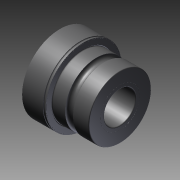
# Autodesk Inventor part: NKXZ12
Saved by Autodesk Inventor 2011 SP1 (Build 150282100, 282)
## iProperties
Created: 2016-11-09
Part Number: NKXZ12
Catalog Web Link: www.cadenas.de
Description: NKXZ-Needle Roller Bearings with Thrust Ball Bearings - With Inner Ring
Vendor: MISUMI
Document SubType Name: Modeling
Designer: psAdmin
Manufacturer: MISUMI
Mass: 8.94729 g
Surface Area: 40.7906 cm^2
Volume: 8.94729 cm^3
Density: 1 g/cm^3
Category: PARTsolutions
Company: MISUMI
Title: NKXZ12
Author: Cadenas PARTsolutions
Comments: Needle Roller Bearings with Thrust Ball Bearings - With Inner Ring
PSOL_IDENT_0: {$CADENAS_DATA\23d-libs\misumi\metric\12_bearing_holders\nkxz.prj},152 {VTYP=3D},{NB=NKXZ12},{LINA=N
PSOL_IDENT_1: KXZ12},{NN=NKXZ},{DATE=17.06.2016 05:47:22},{GEOMDATE=25.02.2016 05:06:56},{VERSION=},{LINEID=30},{L
PSOL_IDENT_2: INESUBID=-1},{WBVAR=}  {NB=NKXZ12},{LINA=NKXZ12},{KT=DUMMY},{PN=NKXZ12},{TYPE=NKXZ},{DD=12},{D=24},{
PSOL_IDENT_3: B=16},{L=23},{T=9},{RR=0.3},{RR1=0.3},{DD1=15},{D1=29.0},{LL=6.5},{AA=23.7}
NN: NKXZ
NT: Needle Roller Bearings with Thrust Ball Bearings - With Inner Ring
NB: NKXZ12
NBSYN: $PN.
LINA: NKXZ12
PN: NKXZ12
DD: 12
D: 24
B: 16
L: 23
T: 9
RR: 0.3
RR1: 0.3
DD1: 15
D1: 29.0
LL: 6.5
AA: 23.7
SUPPLIER: MISUMI
ARTICLENO: NKXZ12
BOMINFO: NKXZ12
CREATOR: CADENAS GmbH
Autodesk Inventor part; units mm, degrees
ref_plane "YZ Plane" through (0, 0, 0) normal (1, 0, 0) x (0, 1, 0)
ref_plane "XZ Plane" through (0, 0, 0) normal (0, 1, 0) x (-1, 0, 0)
ref_plane "XY Plane" through (0, 0, 0) normal (0, 0, 1) x (1, 0, 0)
sketch "Sketch_1" plane through (0, 0, 0) normal (0, 0, 1) x (1, 0, 0)
  line L0 (23, 0) -> (0, 0)
  line L1 (0, 14.5) -> (0, 11.87)
  arc A0 (0, 11.83) -> (0, 11.87) centre (0, 11.85) ccw
  line L2 (0, 11.83) -> (0, 7.8)
  arc A1 (0, 7.8) -> (0.3, 7.5) centre (0.3, 7.8) ccw
  line L3 (0.3, 7.5) -> (7, 7.5)
  line L4 (7, 7.5) -> (7, 6)
  line L5 (7, 6) -> (22.7, 6)
  arc A2 (22.7, 6) -> (23, 6.3) centre (22.7, 6.3) ccw
  line L6 (23, 6.3) -> (23, 7.48)
  arc A3 (23, 7.52) -> (23, 7.48) centre (23, 7.5) ccw
  line L7 (23, 7.52) -> (23, 11.7)
  arc A4 (23, 11.7) -> (22.7, 12) centre (22.7, 11.7) ccw
  line L8 (22.7, 12) -> (17, 12)
  arc A5 (14, 12) -> (17, 12) centre (15.5, 12) ccw
  line L9 (14, 12) -> (9.3, 12)
  arc A6 (9, 12.3) -> (9.3, 12) centre (9, 12) ccw
  line L10 (9, 12.3) -> (9, 14.18)
  arc A7 (9, 14.22) -> (9, 14.18) centre (9, 14.2) ccw
  line L11 (9, 14.22) -> (9, 14.5)
  line L12 (9, 14.5) -> (8.55, 14.5)
  arc A8 (7.95, 14.5) -> (8.55, 14.5) centre (8.25, 14.5) ccw
  line L13 (7.95, 14.5) -> (0, 14.5)
  constraints: 28 end point, 18 point on circle, 9 centre point
revolve "Revolution1" add sketch "Sketch_1" angle 360 about axis through (23, 0, 0) along (1, 0, 0)
ref_plane "to_housing_XY" through (9, 0, 0) normal (1, 0, 0) x (0, 0, -1)
ref_plane "to_housing_YZ" through (9, 0, 0) normal (0, 0, -1) x (0, 1, 0)
ref_plane "to_housing_ZX" through (9, 0, 0) normal (0, 1, 0) x (1, 0, 0)
body "Solid1"
